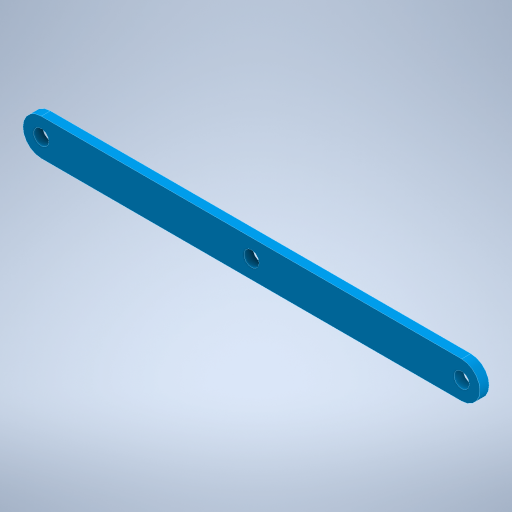
# Autodesk Inventor part: 連桿
Saved by Autodesk Inventor 2023 (Build 270158000, 158)
## iProperties
Created: 2023-03-17
Part Number: 連桿
Material: 一般
Document SubType Name: Modeling
Designer: may9c
Density: 1 g/cm^3
Appearance: 預設
Mass: 0.0815708 g
Surface Area: 1.92987 cm^2
Volume: 0.0815708 cm^3
Author: may9c
Autodesk Inventor part; units mm, degrees
ref_plane "YZ Plane" through (0, 0, 0) normal (1, 0, 0) x (0, 1, 0)
ref_plane "XZ Plane" through (0, 0, 0) normal (0, 1, 0) x (-1, 0, 0)
ref_plane "XY Plane" through (0, 0, 0) normal (0, 0, 1) x (1, 0, 0)
sketch "草圖1" plane through (0, 0, 0) normal (0, 0, 1) x (1, 0, 0)
  line L0 (-69, 0) -> (69, 0) construction
  line L1 (-69, -6) -> (69, -6)
  line L2 (69, 6) -> (-69, 6)
  arc A0 (-69, 6) -> (-69, -6) centre (-69, 0) ccw
  arc A1 (69, -6) -> (69, 6) centre (69, 0) ccw
  circle A2 centre (-69, 0) radius 2.5
  circle A3 centre (0, 0) radius 2.5
  circle A4 centre (69, 0) radius 2.5
  dimension "d0" = 138
  dimension "d1" = 12
  dimension "d2" = 5
  constraints: 8 end point, 5 centre point, 4 coincident, 4 point on circle, 4 tangent, 2 equal radius, 1 horizontal, 1 midpoint, 1 parallel
  measures "d0" distance of L0.end L0.start
  measures "d1" distance between parallel lines of L1 L2
  measures "d2" diameter of A2
extrude "擠出1" add sketch "草圖1" along normal blind 3
